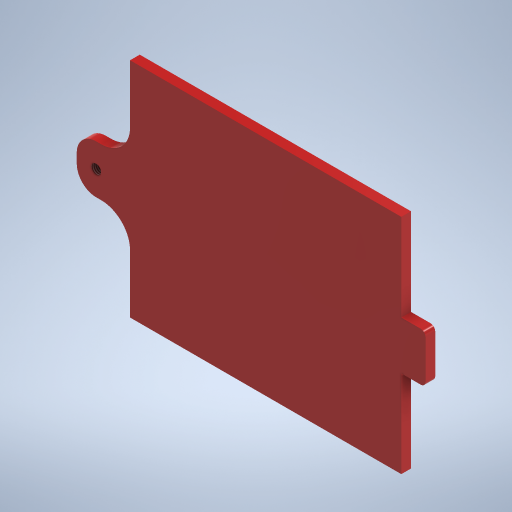
# Autodesk Inventor part: Battery holder lid
Saved by Autodesk Inventor 2023 (Build 270158000, 158)
## iProperties
Created: 2023-12-14
Part Number: Battery holder lid
Material: Generic
Document SubType Name: Modeling
Designer: User
Density: 1 g/cm^3
Appearance: Red
Author: User
Autodesk Inventor part; units mm, degrees
ref_plane "YZ Plane" through (0, 0, 0) normal (1, 0, 0) x (0, 1, 0)
ref_plane "XZ Plane" through (0, 0, 0) normal (0, 1, 0) x (-1, 0, 0)
ref_plane "XY Plane" through (0, 0, 0) normal (0, 0, 1) x (1, 0, 0)
sketch "Sketch1" plane through (0, 0, 0) normal (0, 0, 1) x (1, 0, 0)
  line L0 (57, -1) -> (1, -1)
  line L1 (1, -1) -> (1, -13)
  arc A0 (-5, -19) -> (1, -13) centre (-5, -13) ccw
  line L2 (-5, -19) -> (-6, -19)
  arc A1 (-6, -19) -> (-10, -23) centre (-6, -23) ccw
  line L3 (-10, -23) -> (-10, -25)
  arc A2 (-10, -25) -> (-6, -29) centre (-6, -25) ccw
  line L4 (-6, -29) -> (-5, -29)
  arc A3 (1, -35) -> (-5, -29) centre (-5, -35) ccw
  line L5 (1, -35) -> (1, -47)
  line L6 (1, -47) -> (57, -47)
  line L7 (57, -47) -> (57, -29)
  line L8 (57, -29) -> (61, -29)
  arc A4 (61, -29) -> (62, -28) centre (61, -28) ccw
  line L9 (62, -28) -> (62, -20)
  arc A5 (62, -20) -> (61, -19) centre (61, -20) ccw
  line L10 (61, -19) -> (57, -19)
  line L11 (57, -19) -> (57, -1)
  point P0 (0, 0)
  constraints: 24 end point, 12 point on circle, 7 perpendicular, 6 centre point, 5 parallel
extrude "Extrusion1" add sketch "Sketch1" along normal blind 2
sketch "Sketch2" plane through (0, 0, 2) normal (0, 0, 1) x (1, 0, 0)
  line L0 (-10, -24) -> (-6, -24) construction
  circle A0 centre (-6, -24) radius 1
  line L1 (-10, -24) -> (-6, -24) construction
  point P0 (0, 0)
  point P1 (-10, -23)
  point P2 (-10, -25)
  dimension "d14" = 2
  dimension "d20" = 4
  constraints: 4 end point, 1 centre point, 1 coincident
  measures "d14" diameter of A0
  measures "d20" distance of L0.start L1.end
extrude "Extrusion2" cut sketch "Sketch2" against normal blind 5
thread "Thread1" size "M2x0.4" class "6H" standard "ANSI Metric M Profile" length 10
body "Solid1"
